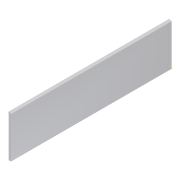
# Autodesk Inventor part: Slidev2
Saved by Autodesk Inventor 2015 (Build 190159000, 159)
## iProperties
Created: 2015-03-13
Part Number: Slidev2
Material: Polycarbonate, Clear
Document SubType Name: Modeling
Designer: Jaden
Density: 1.2 g/cm^3
Appearance: Polycarbonate - Clear
Author: Jaden
Autodesk Inventor part; units mm, degrees
ref_plane "YZ Plane" through (0, 0, 0) normal (1, 0, 0) x (0, 1, 0)
ref_plane "XZ Plane" through (0, 0, 0) normal (0, 1, 0) x (-1, 0, 0)
ref_plane "XY Plane" through (0, 0, 0) normal (0, 0, 1) x (1, 0, 0)
sketch "Sketch1" plane through (0, 0, 0) normal (0, 0, 1) x (1, 0, 0)
  point P0 (0, 0)
sketch "Sketch2" plane through (0, 0, 0) normal (0, 0, 1) x (1, 0, 0)
  line L0 (0, 0) -> (0, 101.6)
  line L1 (0, 0) -> (-6.35, 0)
  line L2 (-6.35, 0) -> (-6.35, 101.6)
  line L3 (0, 101.6) -> (-5.8197, 104.1405)
  line L4 (0, 101.6) -> (6.35, 101.6) construction
  line L5 (-6.35, 101.6) -> (-6.836, 101.8122)
  line L6 (-6.836, 101.8122) -> (-5.8197, 104.1405)
  dimension "d0" = 101.6
  dimension "d1" = 6.35
  dimension "d2" = 6.35
  dimension "d3" = 156.417
  constraints: 14 end point, 2 horizontal, 2 perpendicular, 1 equal length, 1 vertical
  measures "d0" distance of L0.start L0.end
  measures "d1" distance of L0.start L1.end
  measures "d2" distance of L0.end L3.end
  measures "d3" angle of L4 L3
extrude "Extrusion1" add sketch "Sketch2" along normal blind 396.875
body "Solid1"
